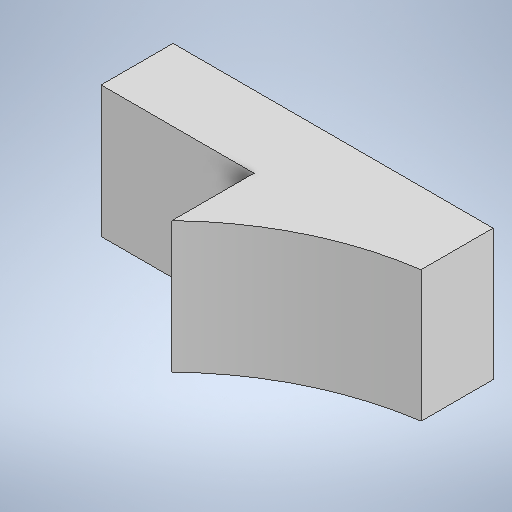
# Autodesk Inventor part: mogo aligner
Saved by Autodesk Inventor 2025.2 (Build 292293000, 293)
## iProperties
Created: 2024-12-10
Part Number: mogo aligner
Material: Generic
Document SubType Name: Modeling
Designer: hmath
Density: 1 g/cm^3
Appearance: Default
Author: hmath
Autodesk Inventor part; units mm, degrees
ref_plane "YZ Plane" through (0, 0, 0) normal (1, 0, 0) x (0, 1, 0)
ref_plane "XZ Plane" through (0, 0, 0) normal (0, 1, 0) x (-1, 0, 0)
ref_plane "XY Plane" through (0, 0, 0) normal (0, 0, 1) x (1, 0, 0)
sketch "Sketch1" plane through (0, 0, 0) normal (0, 0, 1) x (1, 0, 0)
  line L0 (0, 0) -> (52.959, 0)
  line L1 (52.959, 0) -> (52.959, 21.717)
  line L2 (52.959, 21.717) -> (0, 21.717)
  line L3 (0, 21.717) -> (0, 0)
  dimension "d0" = 52.959
  dimension "d1" = 21.717
  constraints: 8 end point, 2 parallel, 1 horizontal, 1 perpendicular
  measures "d0" distance of L1.end L2.end
  measures "d1" distance of L0.end L1.end
extrude "Extrusion1" add sketch "Sketch1" along normal blind 11.9126
sketch "Sketch3" plane through (0, 21.717, 0) normal (0, 1, 0) x (1, 0, 0)
  line L0 (52.959, -11.9126) -> (0, -11.9126) projected
  line L1 (52.959, -11.9126) -> (25.3122, -11.9126)
  line L2 (25.3122, -25.5065) -> (25.3122, -11.9126)
  arc A0 (52.959, -11.9126) -> (25.3122, -25.5065) centre (60.065, -61.2752) ccw
  point P0 (0, 0)
  constraints: 4 end point, 2 point on circle, 1 centre point, 1 perpendicular, 1 point on line
extrude "Extrusion2" add sketch "Sketch3" against normal up to surface (21.717 mm away)
body "Solid1"
